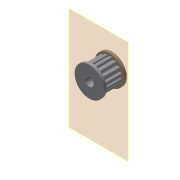
# Autodesk Inventor part: 30_CUBE_openXY_gear_2mmbelt
Saved by Autodesk Inventor 2019 (Build 230136000, 136)
## iProperties
Created: 2020-03-17
Part Number: 30_CUBE_openXY_gear_2mmbelt
Material: Generic
Document SubType Name: Modeling
Designer: diederichbenedict
Density: 1 g/cm^3
Appearance: Default
Author: diederichbenedict
Autodesk Inventor part; units mm, degrees
ref_plane "YZ Plane" through (0, 0, 0) normal (1, 0, 0) x (0, 1, 0)
ref_plane "XZ Plane" through (0, 0, 0) normal (0, 1, 0) x (-1, 0, 0)
ref_plane "XY Plane" through (0, 0, 0) normal (0, 0, 1) x (1, 0, 0)
ref_plane "Work Plane1" through (0, 0, 0) normal (0, 0, 1) x (1, 0, 0)
sketch "Sketch1" plane through (0, 0, 0) normal (0, 0, 1) x (1, 0, 0)
  circle A0 centre (4.149, 7.0628) radius 1.6 projected
  circle A1 centre (4.149, 7.0628) radius 1.6 construction
  line L0 (4.149, 7.0628) -> (4.1493, 3.0628) construction
  arc A2 (3.1573, 3.0949) -> (3.2673, 3.069) centre (4.149, 7.0628) ccw
  arc A3 (3.1377, 3.0998) -> (3.2673, 3.069) centre (4.149, 7.0628) ccw
  arc A4 (5.599, 10.8872) -> (5.3687, 10.9668) centre (4.149, 7.0628) ccw
  arc A5 (7.0291, 9.9668) -> (6.8511, 10.1332) centre (4.149, 7.0628) ccw
  arc A6 (7.0291, 9.9668) -> (6.8511, 10.1332) centre (4.149, 7.0628) ccw
  arc A7 (5.599, 10.8872) -> (5.7734, 10.9392) centre (5.6521, 11.0275) ccw construction
  arc A8 (6.8154, 10.3117) -> (6.8511, 10.1332) centre (6.9502, 10.2458) ccw construction
  arc A9 (5.599, 10.8872) -> (5.7734, 10.9392) centre (5.6521, 11.0275) ccw
  arc A10 (6.8154, 10.3117) -> (6.8511, 10.1332) centre (6.9502, 10.2458) ccw
  arc A11 (6.8154, 10.3117) -> (5.7734, 10.9392) centre (6.3283, 10.6818) ccw
  arc A12 (5.599, 10.8872) -> (6.8511, 10.1332) centre (4.149, 7.0628) ccw
  point P0 (0, 0)
  dimension "d0" = 3.2
  constraints: 23 point on circle, 12 centre point, 4 coincident, 2 concentric, 2 end point, 14 other
  measures "d0" diameter of A1
extrude "Extrusion1" add sketch "Sketch1" along normal blind 6.5
pattern_circular "Circular Pattern1" count 15 over 360 about axis through (4.149, 7.0628, 0) along (0, 0, 1) of "Extrusion1"
sketch "Sketch2" plane through (0, 0, 0) normal (0, 0, -1) x (-1, 0, 0)
  circle A0 centre (-4.149, 7.0628) radius 1.6 projected
  arc A1 (-5.7734, 10.9392) -> (-5.599, 10.8872) centre (-5.6521, 11.0275) ccw projected
  arc A2 (-5.7734, 10.9392) -> (-6.8154, 10.3117) centre (-6.3283, 10.6818) ccw projected
  arc A3 (-6.8511, 10.1332) -> (-6.8154, 10.3117) centre (-6.9502, 10.2458) ccw projected
  arc A4 (-6.8511, 10.1332) -> (-7.0291, 9.9668) centre (-4.149, 7.0628) ccw projected
  arc A5 (-7.2096, 9.9434) -> (-7.0291, 9.9668) centre (-7.1348, 10.0733) ccw projected
  arc A6 (-7.2096, 9.9434) -> (-7.9063, 8.9463) centre (-7.6119, 9.4825) ccw projected
  arc A7 (-7.8663, 8.7687) -> (-7.9063, 8.9463) centre (-8.0026, 8.8313) ccw projected
  arc A8 (-7.8663, 8.7687) -> (-7.9613, 8.5443) centre (-4.149, 7.0628) ccw projected
  arc A9 (-8.1166, 8.4495) -> (-7.9613, 8.5443) centre (-8.1011, 8.5987) ccw projected
  arc A10 (-8.1166, 8.4495) -> (-8.3476, 7.2552) centre (-8.2967, 7.8648) ccw projected
  arc A11 (-8.2388, 7.1093) -> (-8.3476, 7.2552) centre (-8.3888, 7.111) ccw projected
  arc A12 (-8.2388, 7.1093) -> (-8.2343, 6.8657) centre (-4.149, 7.0628) ccw projected
  arc A13 (-8.3376, 6.7158) -> (-8.2343, 6.8657) centre (-8.3841, 6.8584) ccw projected
  arc A14 (-8.3376, 6.7158) -> (-8.0628, 5.5309) centre (-8.2643, 6.1085) ccw projected
  arc A15 (-7.9041, 5.4418) -> (-8.0628, 5.5309) centre (-8.0418, 5.3824) ccw projected
  arc A16 (-7.9041, 5.4418) -> (-7.8009, 5.2211) centre (-4.149, 7.0628) ccw projected
  arc A17 (-7.8344, 5.0422) -> (-7.8009, 5.2211) centre (-7.9348, 5.1536) ccw projected
  arc A18 (-7.8344, 5.0422) -> (-7.1014, 4.0715) centre (-7.5204, 4.5172) ccw projected
  arc A19 (-6.9201, 4.0547) -> (-7.1014, 4.0715) centre (-7.0218, 3.9443) ccw projected
  arc A20 (-6.9201, 4.0547) -> (-6.7361, 3.895) centre (-4.149, 7.0628) ccw projected
  arc A21 (-6.6939, 3.7179) -> (-6.7361, 3.895) centre (-6.831, 3.7788) ccw projected
  arc A22 (-6.6939, 3.7179) -> (-5.6294, 3.1292) centre (-6.1935, 3.366) ccw projected
  arc A23 (-5.457, 3.1876) -> (-5.6294, 3.1292) centre (-5.505, 3.0455) ccw projected
  arc A24 (-5.457, 3.1876) -> (-5.224, 3.1166) centre (-4.149, 7.0628) ccw projected
  arc A25 (-5.1134, 2.972) -> (-5.224, 3.1166) centre (-5.2634, 2.9719) ccw projected
  arc A26 (-5.1134, 2.972) -> (-3.9015, 2.8672) centre (-4.5131, 2.8541) ccw projected
  arc A27 (-3.7678, 2.9906) -> (-3.9015, 2.8672) centre (-3.7538, 2.8413) ccw projected
  arc A28 (-3.7678, 2.9906) -> (-3.526, 3.0206) centre (-4.149, 7.0628) ccw projected
  arc A29 (-3.3661, 2.9335) -> (-3.526, 3.0206) centre (-3.5031, 2.8723) ccw projected
  arc A30 (-3.3661, 2.9335) -> (-2.2164, 3.3306) centre (-2.7698, 3.0699) ccw projected
  arc A31 (-2.1444, 3.4978) -> (-2.2164, 3.3306) centre (-2.0709, 3.367) ccw projected
  arc A32 (-2.1444, 3.4978) -> (-1.9357, 3.6235) centre (-4.149, 7.0628) ccw projected
  arc A33 (-1.7543, 3.6089) -> (-1.9357, 3.6235) centre (-1.8545, 3.4973) ccw projected
  arc A34 (-1.7543, 3.6089) -> (-0.8655, 4.4393) centre (-1.265, 3.9761) ccw projected
  arc A35 (-0.8677, 4.6213) -> (-0.8655, 4.4393) centre (-0.7474, 4.5318) ccw projected
  arc A36 (-0.8677, 4.6213) -> (-0.7281, 4.8211) centre (-4.149, 7.0628) ccw projected
  arc A37 (-0.5565, 4.8816) -> (-0.7281, 4.8211) centre (-0.6027, 4.7389) ccw projected
  arc A38 (-0.5565, 4.8816) -> (-0.0823, 6.0017) centre (-0.2588, 5.416) ccw projected
  arc A39 (-0.1583, 6.1671) -> (-0.0823, 6.0017) centre (-0.012, 6.1342) ccw projected
  arc A40 (-0.1583, 6.1671) -> (-0.1121, 6.4063) centre (-4.149, 7.0628) ccw projected
  arc A41 (0.0201, 6.5314) -> (-0.1121, 6.4063) centre (0.036, 6.3822) ccw projected
  arc A42 (0.0201, 6.5314) -> (-0.0023, 7.7476) centre (0.0747, 7.1407) ccw projected
  arc A43 (-0.139, 7.8677) -> (-0.0023, 7.7476) centre (0.008, 7.8972) ccw projected
  arc A44 (-0.139, 7.8677) -> (-0.1941, 8.105) centre (-4.149, 7.0628) ccw projected
  arc A45 (-0.1241, 8.2731) -> (-0.1941, 8.105) centre (-0.049, 8.1433) ccw projected
  arc A46 (-0.1241, 8.2731) -> (-0.6393, 9.375) centre (-0.3221, 8.8519) ccw projected
  arc A47 (-0.8131, 9.4291) -> (-0.6393, 9.375) centre (-0.6907, 9.5159) ccw projected
  arc A48 (-0.8131, 9.4291) -> (-0.9599, 9.6236) centre (-4.149, 7.0628) ccw projected
  arc A49 (-0.9644, 9.8055) -> (-0.9599, 9.6236) centre (-0.8429, 9.7175) ccw projected
  arc A50 (-0.9644, 9.8055) -> (-1.8832, 10.6027) centre (-1.3807, 10.2538) ccw projected
  arc A51 (-2.0639, 10.5814) -> (-1.8832, 10.6027) centre (-1.9875, 10.7105) ccw projected
  arc A52 (-2.0639, 10.5814) -> (-2.2772, 10.6993) centre (-4.149, 7.0628) ccw projected
  arc A53 (-2.3553, 10.8637) -> (-2.2772, 10.6993) centre (-2.2085, 10.8327) ccw projected
  arc A54 (-2.3553, 10.8637) -> (-3.5188, 11.2182) centre (-2.9179, 11.1039) ccw projected
  arc A55 (-3.6753, 11.1253) -> (-3.5188, 11.2182) centre (-3.658, 11.2743) ccw projected
  arc A56 (-3.6753, 11.1253) -> (-3.9181, 11.1463) centre (-4.149, 7.0628) ccw projected
  arc A57 (-4.0563, 11.2647) -> (-3.9181, 11.1463) centre (-3.9096, 11.2961) ccw projected
  arc A58 (-4.0563, 11.2647) -> (-5.2635, 11.1153) centre (-4.668, 11.2553) ccw projected
  arc A59 (-5.3687, 10.9668) -> (-5.2635, 11.1153) centre (-5.4134, 11.1099) ccw projected
  arc A60 (-5.3687, 10.9668) -> (-5.599, 10.8872) centre (-4.149, 7.0628) ccw projected
  circle A61 centre (-4.149, 7.0628) radius 5.5
  point P0 (0, 0)
  dimension "d10" = 11
  constraints: 1 centre point, 1 coincident
  measures "d10" diameter of A61
extrude "Extrusion2" add sketch "Sketch2" along normal blind 1 contours A1 A60 A59 A58 A57 A56 A55 A54 A53 A52 A51 A50 A49 A48 A47 A46 A45 A44 A43 A42 A41 A40 A39 A38 A37 A36 A35 A34 A33 A32 A31 A30 A29 A28 A27 A26 A25 A24 A23 A22 A21 A20 A19 A18 A17 A16 A15 A14 A13 A12 A11 A10 A9 A8 A7 A6 A5 A4 A3 A2 | A61
sketch "Sketch3" plane through (0, 0, 6.5) normal (0, 0, 1) x (1, 0, 0)
  circle A0 centre (4.149, 7.0628) radius 1.6 projected
  arc A1 (6.8154, 10.3117) -> (6.8511, 10.1332) centre (6.9502, 10.2458) ccw projected
  arc A2 (6.8154, 10.3117) -> (5.7734, 10.9392) centre (6.3283, 10.6818) ccw projected
  arc A3 (5.599, 10.8872) -> (5.7734, 10.9392) centre (5.6521, 11.0275) ccw projected
  arc A4 (5.599, 10.8872) -> (5.3687, 10.9668) centre (4.149, 7.0628) ccw projected
  arc A5 (5.2635, 11.1153) -> (5.3687, 10.9668) centre (5.4134, 11.1099) ccw projected
  arc A6 (5.2635, 11.1153) -> (4.0563, 11.2647) centre (4.668, 11.2553) ccw projected
  arc A7 (3.9181, 11.1463) -> (4.0563, 11.2647) centre (3.9096, 11.2961) ccw projected
  arc A8 (3.9181, 11.1463) -> (3.6753, 11.1253) centre (4.149, 7.0628) ccw projected
  arc A9 (3.5188, 11.2182) -> (3.6753, 11.1253) centre (3.658, 11.2743) ccw projected
  arc A10 (3.5188, 11.2182) -> (2.3553, 10.8637) centre (2.9179, 11.1039) ccw projected
  arc A11 (2.2772, 10.6993) -> (2.3553, 10.8637) centre (2.2085, 10.8327) ccw projected
  arc A12 (2.2772, 10.6993) -> (2.0639, 10.5814) centre (4.149, 7.0628) ccw projected
  arc A13 (1.8832, 10.6027) -> (2.0639, 10.5814) centre (1.9875, 10.7105) ccw projected
  arc A14 (1.8832, 10.6027) -> (0.9644, 9.8055) centre (1.3807, 10.2538) ccw projected
  arc A15 (0.9599, 9.6236) -> (0.9644, 9.8055) centre (0.8429, 9.7175) ccw projected
  arc A16 (0.9599, 9.6236) -> (0.8131, 9.4291) centre (4.149, 7.0628) ccw projected
  arc A17 (0.6393, 9.375) -> (0.8131, 9.4291) centre (0.6907, 9.5159) ccw projected
  arc A18 (0.6393, 9.375) -> (0.1241, 8.2731) centre (0.3221, 8.8519) ccw projected
  arc A19 (0.1941, 8.105) -> (0.1241, 8.2731) centre (0.049, 8.1433) ccw projected
  arc A20 (0.1941, 8.105) -> (0.139, 7.8677) centre (4.149, 7.0628) ccw projected
  arc A21 (0.0023, 7.7476) -> (0.139, 7.8677) centre (-0.008, 7.8972) ccw projected
  arc A22 (0.0023, 7.7476) -> (-0.0201, 6.5314) centre (-0.0747, 7.1407) ccw projected
  arc A23 (0.1121, 6.4063) -> (-0.0201, 6.5314) centre (-0.036, 6.3822) ccw projected
  arc A24 (0.1121, 6.4063) -> (0.1583, 6.1671) centre (4.149, 7.0628) ccw projected
  arc A25 (0.0823, 6.0017) -> (0.1583, 6.1671) centre (0.012, 6.1342) ccw projected
  arc A26 (0.0823, 6.0017) -> (0.5565, 4.8816) centre (0.2588, 5.416) ccw projected
  arc A27 (0.7281, 4.8211) -> (0.5565, 4.8816) centre (0.6027, 4.7389) ccw projected
  arc A28 (0.7281, 4.8211) -> (0.8677, 4.6213) centre (4.149, 7.0628) ccw projected
  arc A29 (0.8655, 4.4393) -> (0.8677, 4.6213) centre (0.7474, 4.5318) ccw projected
  arc A30 (0.8655, 4.4393) -> (1.7543, 3.6089) centre (1.265, 3.9761) ccw projected
  arc A31 (1.9357, 3.6235) -> (1.7543, 3.6089) centre (1.8545, 3.4973) ccw projected
  arc A32 (1.9357, 3.6235) -> (2.1444, 3.4978) centre (4.149, 7.0628) ccw projected
  arc A33 (2.2164, 3.3306) -> (2.1444, 3.4978) centre (2.0709, 3.367) ccw projected
  arc A34 (2.2164, 3.3306) -> (3.3661, 2.9335) centre (2.7698, 3.0699) ccw projected
  arc A35 (3.526, 3.0206) -> (3.3661, 2.9335) centre (3.5031, 2.8723) ccw projected
  arc A36 (3.526, 3.0206) -> (3.7678, 2.9906) centre (4.149, 7.0628) ccw projected
  arc A37 (3.9015, 2.8672) -> (3.7678, 2.9906) centre (3.7538, 2.8413) ccw projected
  arc A38 (3.9015, 2.8672) -> (5.1134, 2.972) centre (4.5131, 2.8541) ccw projected
  arc A39 (5.224, 3.1166) -> (5.1134, 2.972) centre (5.2634, 2.9719) ccw projected
  arc A40 (5.224, 3.1166) -> (5.457, 3.1876) centre (4.149, 7.0628) ccw projected
  arc A41 (5.6294, 3.1292) -> (5.457, 3.1876) centre (5.505, 3.0455) ccw projected
  arc A42 (5.6294, 3.1292) -> (6.6939, 3.7179) centre (6.1935, 3.366) ccw projected
  arc A43 (6.7361, 3.895) -> (6.6939, 3.7179) centre (6.831, 3.7788) ccw projected
  arc A44 (6.7361, 3.895) -> (6.9201, 4.0547) centre (4.149, 7.0628) ccw projected
  arc A45 (7.1014, 4.0715) -> (6.9201, 4.0547) centre (7.0218, 3.9443) ccw projected
  arc A46 (7.1014, 4.0715) -> (7.8344, 5.0422) centre (7.5204, 4.5172) ccw projected
  arc A47 (7.8009, 5.2211) -> (7.8344, 5.0422) centre (7.9348, 5.1536) ccw projected
  arc A48 (7.8009, 5.2211) -> (7.9041, 5.4418) centre (4.149, 7.0628) ccw projected
  arc A49 (8.0628, 5.5309) -> (7.9041, 5.4418) centre (8.0418, 5.3824) ccw projected
  arc A50 (8.0628, 5.5309) -> (8.3376, 6.7158) centre (8.2643, 6.1085) ccw projected
  arc A51 (8.2343, 6.8657) -> (8.3376, 6.7158) centre (8.3841, 6.8584) ccw projected
  arc A52 (8.2343, 6.8657) -> (8.2388, 7.1093) centre (4.149, 7.0628) ccw projected
  arc A53 (8.3476, 7.2552) -> (8.2388, 7.1093) centre (8.3888, 7.111) ccw projected
  arc A54 (8.3476, 7.2552) -> (8.1166, 8.4495) centre (8.2967, 7.8648) ccw projected
  arc A55 (7.9613, 8.5443) -> (8.1166, 8.4495) centre (8.1011, 8.5987) ccw projected
  arc A56 (7.9613, 8.5443) -> (7.8663, 8.7687) centre (4.149, 7.0628) ccw projected
  arc A57 (7.9063, 8.9463) -> (7.8663, 8.7687) centre (8.0026, 8.8313) ccw projected
  arc A58 (7.9063, 8.9463) -> (7.2096, 9.9434) centre (7.6119, 9.4825) ccw projected
  arc A59 (7.0291, 9.9668) -> (7.2096, 9.9434) centre (7.1348, 10.0733) ccw projected
  arc A60 (7.0291, 9.9668) -> (6.8511, 10.1332) centre (4.149, 7.0628) ccw projected
  circle A61 centre (4.149, 7.0628) radius 5.5 projected
  arc A62 (3.9181, 11.1463) -> (4.0563, 11.2647) centre (3.9096, 11.2961) ccw projected
  arc A63 (5.2635, 11.1153) -> (4.0563, 11.2647) centre (4.668, 11.2553) ccw projected
  arc A64 (5.2635, 11.1153) -> (5.3687, 10.9668) centre (5.4134, 11.1099) ccw projected
  arc A65 (5.599, 10.8872) -> (5.3687, 10.9668) centre (4.149, 7.0628) ccw projected
  arc A66 (5.599, 10.8872) -> (5.7734, 10.9392) centre (5.6521, 11.0275) ccw projected
  arc A67 (6.8154, 10.3117) -> (5.7734, 10.9392) centre (6.3283, 10.6818) ccw projected
  arc A68 (6.8154, 10.3117) -> (6.8511, 10.1332) centre (6.9502, 10.2458) ccw projected
  arc A69 (7.0291, 9.9668) -> (6.8511, 10.1332) centre (4.149, 7.0628) ccw projected
  arc A70 (7.0291, 9.9668) -> (7.2096, 9.9434) centre (7.1348, 10.0733) ccw projected
  arc A71 (7.9063, 8.9463) -> (7.2096, 9.9434) centre (7.6119, 9.4825) ccw projected
  arc A72 (7.9063, 8.9463) -> (7.8663, 8.7687) centre (8.0026, 8.8313) ccw projected
  arc A73 (7.9613, 8.5443) -> (7.8663, 8.7687) centre (4.149, 7.0628) ccw projected
  arc A74 (7.9613, 8.5443) -> (8.1166, 8.4495) centre (8.1011, 8.5987) ccw projected
  arc A75 (8.3476, 7.2552) -> (8.1166, 8.4495) centre (8.2967, 7.8648) ccw projected
  arc A76 (8.3476, 7.2552) -> (8.2388, 7.1093) centre (8.3888, 7.111) ccw projected
  arc A77 (8.2343, 6.8657) -> (8.2388, 7.1093) centre (4.149, 7.0628) ccw projected
  arc A78 (8.2343, 6.8657) -> (8.3376, 6.7158) centre (8.3841, 6.8584) ccw projected
  arc A79 (8.0628, 5.5309) -> (8.3376, 6.7158) centre (8.2643, 6.1085) ccw projected
  arc A80 (8.0628, 5.5309) -> (7.9041, 5.4418) centre (8.0418, 5.3824) ccw projected
  arc A81 (7.8009, 5.2211) -> (7.9041, 5.4418) centre (4.149, 7.0628) ccw projected
  arc A82 (7.8009, 5.2211) -> (7.8344, 5.0422) centre (7.9348, 5.1536) ccw projected
  arc A83 (7.1014, 4.0715) -> (7.8344, 5.0422) centre (7.5204, 4.5172) ccw projected
  arc A84 (7.1014, 4.0715) -> (6.9201, 4.0547) centre (7.0218, 3.9443) ccw projected
  arc A85 (6.7361, 3.895) -> (6.9201, 4.0547) centre (4.149, 7.0628) ccw projected
  arc A86 (6.7361, 3.895) -> (6.6939, 3.7179) centre (6.831, 3.7788) ccw projected
  arc A87 (5.6294, 3.1292) -> (6.6939, 3.7179) centre (6.1935, 3.366) ccw projected
  arc A88 (5.6294, 3.1292) -> (5.457, 3.1876) centre (5.505, 3.0455) ccw projected
  arc A89 (5.224, 3.1166) -> (5.457, 3.1876) centre (4.149, 7.0628) ccw projected
  arc A90 (5.224, 3.1166) -> (5.1134, 2.972) centre (5.2634, 2.9719) ccw projected
  arc A91 (3.9015, 2.8672) -> (5.1134, 2.972) centre (4.5131, 2.8541) ccw projected
  arc A92 (3.9015, 2.8672) -> (3.7678, 2.9906) centre (3.7538, 2.8413) ccw projected
  arc A93 (3.526, 3.0206) -> (3.7678, 2.9906) centre (4.149, 7.0628) ccw projected
  arc A94 (3.526, 3.0206) -> (3.3661, 2.9335) centre (3.5031, 2.8723) ccw projected
  arc A95 (2.2164, 3.3306) -> (3.3661, 2.9335) centre (2.7698, 3.0699) ccw projected
  arc A96 (2.2164, 3.3306) -> (2.1444, 3.4978) centre (2.0709, 3.367) ccw projected
  arc A97 (1.9357, 3.6235) -> (2.1444, 3.4978) centre (4.149, 7.0628) ccw projected
  arc A98 (1.9357, 3.6235) -> (1.7543, 3.6089) centre (1.8545, 3.4973) ccw projected
  arc A99 (0.8655, 4.4393) -> (1.7543, 3.6089) centre (1.265, 3.9761) ccw projected
  arc A100 (0.8655, 4.4393) -> (0.8677, 4.6213) centre (0.7474, 4.5318) ccw projected
  arc A101 (0.7281, 4.8211) -> (0.8677, 4.6213) centre (4.149, 7.0628) ccw projected
  arc A102 (0.7281, 4.8211) -> (0.5565, 4.8816) centre (0.6027, 4.7389) ccw projected
  arc A103 (0.0823, 6.0017) -> (0.5565, 4.8816) centre (0.2588, 5.416) ccw projected
  arc A104 (0.0823, 6.0017) -> (0.1583, 6.1671) centre (0.012, 6.1342) ccw projected
  arc A105 (0.1121, 6.4063) -> (0.1583, 6.1671) centre (4.149, 7.0628) ccw projected
  arc A106 (0.1121, 6.4063) -> (-0.0201, 6.5314) centre (-0.036, 6.3822) ccw projected
  arc A107 (0.0023, 7.7476) -> (-0.0201, 6.5314) centre (-0.0747, 7.1407) ccw projected
  arc A108 (0.0023, 7.7476) -> (0.139, 7.8677) centre (-0.008, 7.8972) ccw projected
  arc A109 (0.1941, 8.105) -> (0.139, 7.8677) centre (4.149, 7.0628) ccw projected
  arc A110 (0.1941, 8.105) -> (0.1241, 8.2731) centre (0.049, 8.1433) ccw projected
  arc A111 (0.6393, 9.375) -> (0.1241, 8.2731) centre (0.3221, 8.8519) ccw projected
  arc A112 (0.6393, 9.375) -> (0.8131, 9.4291) centre (0.6907, 9.5159) ccw projected
  arc A113 (0.9599, 9.6236) -> (0.8131, 9.4291) centre (4.149, 7.0628) ccw projected
  arc A114 (0.9599, 9.6236) -> (0.9644, 9.8055) centre (0.8429, 9.7175) ccw projected
  arc A115 (1.8832, 10.6027) -> (0.9644, 9.8055) centre (1.3807, 10.2538) ccw projected
  arc A116 (1.8832, 10.6027) -> (2.0639, 10.5814) centre (1.9875, 10.7105) ccw projected
  arc A117 (2.2772, 10.6993) -> (2.0639, 10.5814) centre (4.149, 7.0628) ccw projected
  arc A118 (2.2772, 10.6993) -> (2.3553, 10.8637) centre (2.2085, 10.8327) ccw projected
  arc A119 (3.5188, 11.2182) -> (2.3553, 10.8637) centre (2.9179, 11.1039) ccw projected
  arc A120 (3.5188, 11.2182) -> (3.6753, 11.1253) centre (3.658, 11.2743) ccw projected
  arc A121 (3.9181, 11.1463) -> (3.6753, 11.1253) centre (4.149, 7.0628) ccw projected
  point P0 (0, 0)
extrude "Extrusion3" add sketch "Sketch3" along normal blind 1 contours A1 A60 A59 A58 A57 A56 A55 A54 A53 A52 A51 A50 A49 A48 A47 A46 A45 A44 A43 A42 A41 A40 A39 A38 A37 A36 A35 A34 A33 A32 A31 A30 A29 A28 A27 A26 A25 A24 A23 A22 A21 A20 A19 A18 A17 A16 A15 A14 A13 A12 A11 A10 A9 A8 A7 A6 A5 A4 A3 A2 | A61
body "Solid1"
